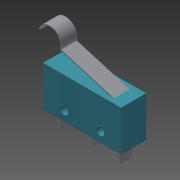
# Autodesk Inventor part: EndStopSwitch
Saved by Autodesk Inventor 2014 SP1 (Build 180222100, 222)
## iProperties
Created: 2014-03-02
Part Number: EndStopSwitch
Material: ABS Plastic
Document SubType Name: Modeling
Designer: Jack
Density: 1.06 g/cm^3
Appearance: Cadet Blue
Author: Jack
Autodesk Inventor part; units mm, degrees
ref_plane "YZ Plane" through (0, 0, 0) normal (1, 0, 0) x (0, 1, 0)
ref_plane "XZ Plane" through (0, 0, 0) normal (0, 1, 0) x (-1, 0, 0)
ref_plane "XY Plane" through (0, 0, 0) normal (0, 0, 1) x (1, 0, 0)
sketch "Sketch1" plane through (0, 0, 0) normal (0, 1, 0) x (-1, 0, 0)
  line L0 (0, 0) -> (19.8, 0)
  line L1 (19.8, 0) -> (19.8, 10.3)
  line L2 (19.8, 10.3) -> (0, 10.3)
  line L3 (0, 10.3) -> (0, 0)
  dimension "d0" = 19.8
  dimension "d1" = 10.3
  constraints: 8 end point, 2 perpendicular, 1 horizontal, 1 parallel
  measures "d0" distance of L0.start L0.end
  measures "d1" distance of L0.end L1.end
extrude "Extrusion1" add sketch "Sketch1" along normal blind 6.4
sketch "Sketch2" plane through (0, 6.4, 0) normal (0, 1, 0) x (1, 0, 0)
  line L0 (0, 0) -> (-19.8, 0) projected
  line L1 (-19.8, 0) -> (-19.8, -10.3) projected
  circle A0 centre (-14.5, -2.5) radius 1
  circle A1 centre (-5.3, -2.5) radius 1
  dimension "d4" = 2
  dimension "d5" = 2
  dimension "d6" = 9.2
  dimension "d7" = 2.5
  dimension "d8" = 5.3
  constraints: 2 centre point, 1 horizontal alignment
  measures "d4" diameter of A0
  measures "d5" diameter of A1
  measures "d6" distance of A0.centre A1.centre
  measures "d7" distance from line of L0 A0.centre
  measures "d8" distance from line of L1 A0.centre
extrude "Extrusion2" cut sketch "Sketch2" against normal blind 6.6
sketch "Sketch3" plane through (0, 0, 0) normal (0, 0, -1) x (-1, 0, 0)
  line L0 (0, 0) -> (19.8, 0) projected
  line L1 (19.8, 0) -> (19.8, 6.4) projected
  line L2 (0, 0) -> (0, 6.4) projected
  line L3 (17.3, 4.7) -> (17.8, 4.7)
  line L4 (17.8, 4.7) -> (17.8, 1.7)
  line L5 (17.8, 1.7) -> (17.3, 1.7)
  line L6 (17.3, 1.7) -> (17.3, 4.7)
  line L7 (9.25, 4.7) -> (9.75, 4.7)
  line L8 (9.75, 4.7) -> (9.75, 1.7)
  line L9 (9.75, 1.7) -> (9.25, 1.7)
  line L10 (9.25, 1.7) -> (9.25, 4.7)
  line L11 (2, 4.7) -> (2.5, 4.7)
  line L12 (2.5, 4.7) -> (2.5, 1.7)
  line L13 (2.5, 1.7) -> (2, 1.7)
  line L14 (2, 1.7) -> (2, 4.7)
  dimension "d11" = 0.5
  dimension "d12" = 3
  dimension "d13" = 0.5
  dimension "d14" = 3
  dimension "d15" = 0.5
  dimension "d16" = 3
  dimension "d17" = 1.7
  dimension "d18" = 2
  dimension "d19" = 2
  dimension "d20" = 7.25
  constraints: 24 end point, 6 parallel, 4 perpendicular, 2 horizontal alignment
  measures "d11" distance of L3.start L3.end
  measures "d12" distance of L3.end L4.end
  measures "d13" distance of L10.end L7.end
  measures "d14" distance of L7.end L8.end
  measures "d15" distance of L14.end L11.end
  measures "d16" distance of L11.end L12.end
  measures "d17" distance between parallel lines of L0 L5
  measures "d18" distance between parallel lines of L2 L14
  measures "d19" distance between parallel lines of L1 L4
  measures "d20" distance between parallel lines of L12 L8
extrude "Extrusion3" add sketch "Sketch3" along normal blind 4
ref_plane "Work Plane1" through (0, 5.2, 0) normal (0, 1, 0) x (1, 0, 0)
sketch "Sketch4" plane through (0, 5.2, 0) normal (0, 1, 0) x (1, 0, 0)
  circle A0 centre (-14.5, -2.5) radius 1 projected
  circle A1 centre (-5.3, -2.5) radius 1 projected
  line L0 (0, 0) -> (-19.8, 0) projected
  line L1 (-19.8, 0) -> (-19.8, -10.3) projected
  line L2 (-19.8, -10.3) -> (0, -10.3) projected
  line L3 (0, -10.3) -> (0, 0) projected
  line L4 (-3, -10.3) -> (-16.4164, -14.3)
  arc A2 (-22.1663, -16.0143) -> (-16.4164, -14.3) centre (-19.2914, -15.1571) ccw
  line L5 (-3.0857, -10.0125) -> (-16.8056, -14.103)
  arc A3 (-21.8788, -15.9286) -> (-16.8056, -14.103) centre (-19.2914, -15.1571) ccw
  line L6 (-21.8788, -15.9286) -> (-22.1663, -16.0143)
  line L7 (-4.05, -10.3) -> (-3, -10.3)
  dimension "d25" = 3
  dimension "d26" = 6
  dimension "d27" = 3
  dimension "d28" = 4
  dimension "d29" = 20
  dimension "d30" = 0.3
  constraints: 8 end point, 4 point on circle, 4 point on line, 2 centre point, 1 collinear, 1 parallel, 1 other
  measures "d25" distance from line of L3 L4.start
  measures "d26" distance of L4.end L6.end
  measures "d27" radius of A2
  measures "d28" distance from line of L2 L4.end
  measures "d29" distance of L6.end L4.start
  measures "d30" distance between parallel lines of L4 L5
extrude "Extrusion4" add sketch "Sketch4" against normal blind 4 contours L4 A2 L6 A3 L5 L2
body "Solid1"
